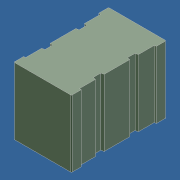
# Autodesk Inventor part: M20121S3A1G13BR-switch
Saved by Autodesk Inventor 2014 (Build 180170000, 170)
## iProperties
Category: PARTsolutions
Created: 2013-12-29
Part Number: M20121S3A1G13BR-switch
Catalog Web Link: www.cadenas.de
Description: Bracket Mount Miniature Toggles - Switch - Series M - Miniature Toggles
Document SubType Name: Modeling
Designer: PARTsolutions
Material: Generic
Density: 1 g/cm^3
Appearance: RGB(78,110,71)
NB: M20121S3A1G13BR-switch
NN: Bracket Mount Miniature Toggles - Switch
NT: Series M - Miniature Toggles
NBSYN: $PN.-switch
LINA: M20121S3A1G13BR-switch
PN: M20121S3A1G13BR
SRS: M20
PLS: 1
CRCTSALG: '2','2 - ON/NONE/ON','3','3 - ON/OFF/ON','5','5 - ON/NONE/(ON)','8','8 - (ON)/OFF/(ON)','9','9 - ON/OFF/(ON)','4', '4 - ON/ON/ON','6','6 - (ON)/ON/(ON)','7','7 - ON/ON/(ON)'
CRCTS: 2
TGGL: 1
TGGLSALG: 'S', 'S - .413" (10.5mm) Bat','S2', 'S2 - .200" (5.08mm) Bat','S3', 'S3 - .256" (6.5mm) Bat','E', 'E - .450" (11.4mm) Flatted','E2', 'E2 - .256" (6.5mm) Flatted','E4', 'E4 - .840" (21.3mm) Flatted','Q', 'Q - .550" (14.0mm) Cone','Q2', 'Q2 - .640" (16.26mm) Cone','Q4', 'Q4 - .840" (21.3mm) Cone'
TGGLS: S3
BSHNGALG: 'A2', 'A2 - .280" (7.1mm) Smooth with Keyway','S2', 'S2 - .350" (8.9mm) Smooth with Keyway','A1', 'A1 - .280" (7.1mm) Threaded with Keyway','S1', 'S1 - .350" (8.9mm) Threaded with Keyway'
BSHNG: A1
CMR: G
TRMNLSALG: '13','13 - .250" (6.35mm) Straight PC with .465" (11.8mm) Bracket','15','15 - .425" (10.8mm) Straight PC with .630" (16.0mm) Bracket','17','17 - .964" (24.5mm) Straight PC with 1.150" (29.2mm) Bracket','23', '23 - .250" (6.35mm) Straight PC with .465" (11.8mm) Reinforced Bracket','25', '25 - .425" (10.8mm) Straight PC with .630" (16.0mm) Reinforced Bracket','26', '26 - .750" (19.05mm) Straight PC with .953" (24.2mm) Reinforced Bracket'
TRMNLS: 13
CPSALG: '','N/A'
CCLRALG: '','N/A'
WIDTH: 0.512
HEIGHT: 0.371
LENGTH: 0.311
A: 0.000
TRMNLNOH: 1.000
ROTALG: 0.262
ANG: 12.500
TRMNLOV: 3.000
LTRMNL: 0.073
POS: 0.000
BR: B
TRMNLALGSE: 03
KT: DUMMY
SUPPLIER: NKKSWITCHES
ARTICLENO: M20121S3A1G13BR-switch
BOMINFO: M20121S3A1G13BR-switch
CREATOR: CADENAS GmbH
PSOL_IDENT_0: {$CADENAS_DATA\23d-libs\nkkswitches\toggle\m\parts\m_br_switch.prj},266 {VTYP=3D},{NB=M20121S3A1G13B
PSOL_IDENT_1: R-switch},{LINA=M20121S3A1G13BR-switch},{NN=Bracket Mount Miniature Toggles - Switch},{DATE=28.05.20
PSOL_IDENT_2: 13 11:19:09},{GEOMDATE=28.05.2013 12:34:00},{VERSION=},{LINEID=10},{LINESUBID=-1},{WBVAR=PLS,CRCTS,T
PSOL_IDENT_3: GGL,TGGLS,BSHNG,CMR,TRMNLS,CPS,CCLR}  {NB=M20121S3A1G13BR-switch},{LINA=M20121S3A1G13BR-switch},{KT=
PSOL_IDENT_4: DUMMY},{PN=M20121S3A1G13BR},{SRS=M20},{PLS=1},{CRCTSALG='2','2 - ON/NONE/ON','3','3 - ON/OFF/ON','5'
PSOL_IDENT_5: ,'5 - ON/NONE/(ON)','8','8 - (ON)/OFF/(ON)','9','9 - ON/OFF/(ON)','4', '4 - ON/ON/ON','6','6 - (ON)/
PSOL_IDENT_6: ON/(ON)','7','7 - ON/ON/(ON)'},{CRCTS=2},{TGGL=1},{TGGLSALG='S', 'S - .413\" (10.5mm) Bat','S2', 'S2
PSOL_IDENT_7: - .200\" (5.08mm) Bat','S3', 'S3 - .256\" (6.5mm) Bat','E', 'E - .450\" (11.4mm) Flatted','E2', 'E2
PSOL_IDENT_8: - .256\" (6.5mm) Flatted','E4', 'E4 - .840\" (21.3mm) Flatted','Q', 'Q - .550\" (14.0mm) Cone','Q2'
PSOL_IDENT_9: , 'Q2 - .640\" (16.26mm) Cone','Q4', 'Q4 - .840\" (21.3mm) Cone'},{TGGLS=S3},{BSHNGALG='A2', 'A2 - .
PSOL_IDENT_10: 280\" (7.1mm) Smooth with Keyway','S2', 'S2 - .350\" (8.9mm) Smooth with Keyway','A1', 'A1 - .280\"
PSOL_IDENT_11: (7.1mm) Threaded with Keyway','S1', 'S1 - .350\" (8.9mm) Threaded with Keyway'},{BSHNG=A1},{CMR=G},{
PSOL_IDENT_12: TRMNLSALG='13','13 - .250\" (6.35mm) Straight PC with .465\" (11.8mm) Bracket','15','15 - .425\" (10
PSOL_IDENT_13: .8mm) Straight PC with .630\" (16.0mm) Bracket','17','17 - .964\" (24.5mm) Straight PC with 1.150\"
PSOL_IDENT_14: (29.2mm) Bracket','23', '23 - .250\" (6.35mm) Straight PC with .465\" (11.8mm) Reinforced Bracket','
PSOL_IDENT_15: 25', '25 - .425\" (10.8mm) Straight PC with .630\" (16.0mm) Reinforced Bracket','26', '26 - .750\" (
PSOL_IDENT_16: 19.05mm) Straight PC with .953\" (24.2mm) Reinforced Bracket'},{TRMNLS=13},{CPSALG='','N/A'},{CPS=},
PSOL_IDENT_17: {CPSPN=},{CCLRALG='','N/A'},{CCLR=},{DSH=},{WIDTH=0.512},{HEIGHT=0.371},{LENGTH=0.311},{A=0},{TRMNLN
PSOL_IDENT_18: OH=1},{ROTALG=0.2625},{ANG=12.5},{TRMNLOV=3},{LTRMNL=0.073},{POS=0},{BR=B},{TRMNLALGSE=03}
Title: M20121S3A1G13BR-switch
Author: Cadenas PARTsolutions
Comments: Series M - Miniature Toggles
Autodesk Inventor part; units mm, degrees
sketch "Sketch_2" plane through (0, -0.254, 0) normal (0, 1, 0) x (1, 0, 0)
  line L0 (-3.9497, -5.1435) -> (-3.9497, -6.3724)
  arc A0 (-3.9497, -6.3724) -> (-3.8197, -6.5024) centre (-3.8197, -6.3724) ccw
  line L1 (-3.8197, -6.5024) -> (3.8197, -6.5024)
  arc A1 (3.8197, -6.5024) -> (3.9497, -6.3724) centre (3.8197, -6.3724) ccw
  line L2 (3.9497, -6.3724) -> (3.9497, -5.1435)
  line L3 (3.9497, -5.1435) -> (3.6957, -5.1435)
  line L4 (3.6957, -5.1435) -> (3.6957, -2.9397)
  line L5 (3.6957, -2.9397) -> (3.3147, -2.8725)
  line L6 (3.3147, -2.8725) -> (3.3147, -1.8265)
  line L7 (3.3147, -1.8265) -> (3.6957, -1.7593)
  line L8 (3.6957, -1.7593) -> (3.6957, 1.7593)
  line L9 (3.6957, 1.7593) -> (3.3147, 1.8265)
  line L10 (3.3147, 1.8265) -> (3.3147, 2.8725)
  line L11 (3.3147, 2.8725) -> (3.6957, 2.9397)
  line L12 (3.6957, 2.9397) -> (3.6957, 5.1435)
  line L13 (3.6957, 5.1435) -> (3.9497, 5.1435)
  line L14 (3.9497, 5.1435) -> (3.9497, 6.3724)
  arc A2 (3.9497, 6.3724) -> (3.8197, 6.5024) centre (3.8197, 6.3724) ccw
  line L15 (3.8197, 6.5024) -> (-3.8197, 6.5024)
  arc A3 (-3.8197, 6.5024) -> (-3.9497, 6.3724) centre (-3.8197, 6.3724) ccw
  line L16 (-3.9497, 6.3724) -> (-3.9497, 5.1435)
  line L17 (-3.9497, 5.1435) -> (-3.6957, 5.1435)
  line L18 (-3.6957, 5.1435) -> (-3.6957, 2.9397)
  line L19 (-3.6957, 2.9397) -> (-3.3147, 2.8725)
  line L20 (-3.3147, 2.8725) -> (-3.3147, 1.8265)
  line L21 (-3.3147, 1.8265) -> (-3.6957, 1.7593)
  line L22 (-3.6957, 1.7593) -> (-3.6957, -1.7593)
  line L23 (-3.6957, -1.7593) -> (-3.3147, -1.8265)
  line L24 (-3.3147, -1.8265) -> (-3.3147, -2.8725)
  line L25 (-3.3147, -2.8725) -> (-3.6957, -2.9397)
  line L26 (-3.6957, -2.9397) -> (-3.6957, -5.1435)
  line L27 (-3.6957, -5.1435) -> (-3.9497, -5.1435)
  constraints: 56 end point, 8 point on circle, 4 centre point
extrude "Extrusion1" add sketch "Sketch_2" against normal blind 9.1694
sketch "Sketch_1" plane through (0, -9.4234, 0) normal (0, 1, 0) x (1, 0, 0)
  line L0 (-3.1877, 6.1184) -> (-3.1877, -6.1184)
  arc A0 (-3.1877, -6.1184) -> (-3.0577, -6.2484) centre (-3.0577, -6.1184) ccw
  line L1 (-3.0577, -6.2484) -> (3.0577, -6.2484)
  arc A1 (3.0577, -6.2484) -> (3.1877, -6.1184) centre (3.0577, -6.1184) ccw
  line L2 (3.1877, -6.1184) -> (3.1877, 6.1184)
  arc A2 (3.1877, 6.1184) -> (3.0577, 6.2484) centre (3.0577, 6.1184) ccw
  line L3 (3.0577, 6.2484) -> (-3.0577, 6.2484)
  arc A3 (-3.0577, 6.2484) -> (-3.1877, 6.1184) centre (-3.0577, 6.1184) ccw
  constraints: 8 end point, 8 point on circle, 4 centre point
extrude "Extrusion2" cut sketch "Sketch_1" along normal blind 0.0254
sketch "Sketch_7" plane through (0, -9.4234, 0) normal (0, 1, 0) x (1, 0, 0)
  line L0 (-0.9271, 5.0927) -> (-0.9271, 4.3053)
  line L1 (-0.9271, 4.3053) -> (0.9271, 4.3053)
  line L2 (0.9271, 4.3053) -> (0.9271, 5.0927)
  line L3 (0.9271, 5.0927) -> (-0.9271, 5.0927)
  constraints: 8 end point
extrude "Extrusion3" cut sketch "Sketch_7" along normal blind 0.254
pattern_linear "Rectangular Pattern1" count 3 spacing 4.699 along (0, 0, 1) of "Extrusion3"
ref_plane "rot_XY" through (0, 6.6675, 0) normal (1, 0, 0) x (0, 0, -1)
ref_plane "rot_YZ" through (0, 6.6675, 0) normal (0, 0, -1) x (0, 1, 0)
ref_plane "rot_ZX" through (0, 6.6675, 0) normal (0, 1, 0) x (1, 0, 0)
ref_plane "to_cover_XY" through (0, -0.254, 0) normal (0, 1, 0) x (1, 0, 0)
ref_plane "to_cover_YZ" through (0, -0.254, 0) normal (1, 0, 0) x (0, 0, -1)
ref_plane "to_cover_ZX" through (0, -0.254, 0) normal (0, 0, -1) x (0, 1, 0)
ref_plane "to_terminals_XY" through (0, -9.4234, 0) normal (0, 1, 0) x (1, 0, 0)
ref_plane "to_terminals_YZ" through (0, -9.4234, 0) normal (1, 0, 0) x (0, 0, -1)
ref_plane "to_terminals_ZX" through (0, -9.4234, 0) normal (0, 0, -1) x (0, 1, 0)
body "Solid1"
